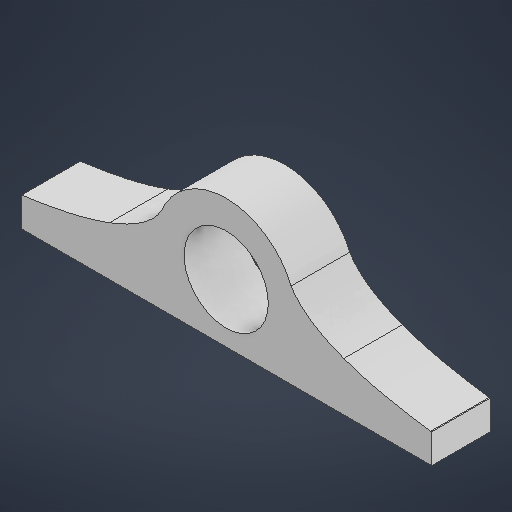
# Autodesk Inventor part: chassis 2
Saved by Autodesk Inventor 2027 (Build 310192060, 192F)
## iProperties
Created: 2026-07-01
Part Number: chassis 2
Material: Generic
Document SubType Name: Modeling
Designer: loren
Density: 1 g/cm^3
Appearance: Default
Author: loren
Autodesk Inventor part; units mm, degrees
ref_plane "YZ Plane" through (0, 0, 0) normal (1, 0, 0) x (0, 1, 0)
ref_plane "XZ Plane" through (0, 0, 0) normal (0, 1, 0) x (-1, 0, 0)
ref_plane "XY Plane" through (0, 0, 0) normal (0, 0, 1) x (1, 0, 0)
sketch "Sketch1" plane through (0, 0, 0) normal (0, 1, 0) x (-1, 0, 0)
  line L0 (-17.5, 2.5) -> (17.5, 2.5)
  line L1 (17.5, 2.5) -> (17.5, -2.5)
  line L2 (17.5, -2.5) -> (-17.5, -2.5)
  line L3 (-17.5, -2.5) -> (-17.5, 2.5)
  line L4 (-17.5, 2.5) -> (17.5, -2.5) construction
  line L5 (17.5, 2.5) -> (-17.5, -2.5) construction
  line L6 (-10, 2.5) -> (10, 2.5)
  line L7 (10, 2.5) -> (10, -2.5)
  line L8 (10, -2.5) -> (-10, -2.5)
  line L9 (-10, -2.5) -> (-10, 2.5)
  line L10 (-10, 2.5) -> (10, -2.5) construction
  line L11 (10, 2.5) -> (-10, -2.5) construction
  point P0 (0, 0)
  dimension "d0" = 35
  dimension "d1" = 5
  dimension "d2" = 20
  constraints: 24 end point, 4 midpoint, 4 parallel, 2 horizontal, 2 perpendicular, 1 point on line
  measures "d0" distance of L1.end L2.end
  measures "d1" distance of L0.end L1.end
  measures "d2" distance of L7.end L8.end
extrude "Extrusion1" add sketch "Sketch1" along normal blind 2.5 contours L0 L9 L2 L3 | L0 L1 L2 L7
extrude "Extrusion2" add sketch "Sketch1" along normal blind 30 contours L0 L7 L2 L9
sketch "Sketch2" plane through (-17.5, 0, 2.5) normal (0, 0, 1) x (1, 0, 0)
  line L0 (0, 2.5) -> (7.5, 2.5) projected
  line L1 (27.5, 2.5) -> (35, 2.5) projected
  line L2 (27.5, 2.5) -> (27.5, 30) projected
  line L3 (7.5, 2.5) -> (7.5, 30) projected
  line L4 (7.5, 30) -> (27.5, 30) projected
  line L5 (35, 0) -> (0, 0) projected
  line L6 (0, 0) -> (0, 2.5) projected
  line L7 (35, 0) -> (35, 2.5) projected
  line L8 (7.5, 2.5) -> (0, 2.5) projected
  line L9 (0, 0) -> (35, 0) projected
  circle A0 centre (17.4535, 4.99) radius 3.595
  circle A1 centre (17.4535, 4.99) radius 6
  line L10 (12.1387, 7.7745) -> (11.4535, 5.8766) construction
  line L11 (11.4535, 5.8766) -> (8.7602, 4.0511) construction
  line L12 (8.7602, 4.0511) -> (4.3576, 3.0847) construction
  line L13 (4.3576, 3.0847) -> (0, 2.5) construction
  spline S0 degree 4 poles (12.1387, 7.7745) (11.4535, 5.8766) (8.7602, 4.0511) (4.3576, 3.0847) (0, 2.5) knots 1 1 1 1 1 2 2 2 2 2
  line L14 (17.4535, 4.99) -> (17.4535, 2.7924)
  line L15 (22.7682, 7.7745) -> (23.4535, 5.8766) construction
  line L16 (23.4535, 5.8766) -> (26.1467, 4.0511) construction
  line L17 (26.1467, 4.0511) -> (30.5493, 3.0847) construction
  line L18 (30.5493, 3.0847) -> (34.907, 2.5) construction
  spline S1 degree 4 poles (22.7682, 7.7745) (23.4535, 5.8766) (26.1467, 4.0511) (30.5493, 3.0847) (34.907, 2.5) knots 1 1 1 1 1 2 2 2 2 2
  point P0 (17.5, 0)
  point P1 (17.5, 0)
  point P2 (17.5, 0)
  point P3 (17.5, 0)
  point P4 (7.5, 10.9282)
  point P5 (27.5, 10.9282)
  point P6 (17.5, 0)
  point P7 (7.5, 6.3541)
  point P8 (27.5, 4.99)
  point P9 (7.5, 6.3541)
  point P10 (7.5, 4.2058)
  point P11 (11.9072, 7.2788)
  point P12 (22.9998, 7.2788)
  point P13 (27.5, 4.171)
  dimension "d77" = 12
  dimension "d58" = 7.19
  dimension "d59" = 4.99
  constraints: 5 point on line, 5 symmetric about line, 3 midpoint, 2 end point, 1 centre point, 1 coincident, 1 vertical, 9 other
  measures "d58" diameter of A0
  measures "d59" vertical distance of A0.centre point (17.5, 0)
extrude "Extrusion10" cut sketch "Sketch2" against normal blind 19.9625 contours A0
sketch "Sketch4" plane through (0, 0, 0) normal (0, -1, 0) x (1, 0, 0)
  line L0 (-17.5, -2.5) -> (-17.5, 2.5) projected
  line L1 (17.5, 2.5) -> (17.5, -2.5) projected
  circle A0 centre (-15, 0) radius 1.25
  line L2 (0, 0) -> (0, -2.2374)
  circle A1 centre (15, 0) radius 1.25
  point P0 (-17.5, 0)
  point P1 (17.5, 0)
  dimension "d68" = 2.5
  dimension "d71" = 2.5
  dimension "d72" = 2.5
  constraints: 2 centre point, 2 end point, 2 midpoint, 1 symmetric about line, 1 vertical, 1 other
  measures "d68" diameter of A0
  measures "d71" distance of point (-17.5, 0) A0.centre
  measures "d72" distance of point (17.5, 0) A1.centre
extrude "Extrusion14" cut sketch "Sketch4" against normal blind 2
extrude "Extrusion17" cut sketch "Sketch2" against normal blind 5 contours L3 L4 L2 S1 A1 S0
extrude "Extrusion18" add sketch "Sketch2" against normal blind 5 contours S0 L3 L0 | S1 L1 L2
body "Solid1"
